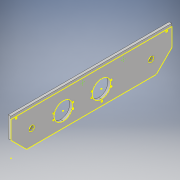
# Autodesk Inventor part: DriveTrainPlate
Saved by Autodesk Inventor 2017 (Build 210142000, 142)
## iProperties
Created: 2016-09-21
Part Number: DriveTrainPlate
Material: Generic
Document SubType Name: Modeling
Designer: RoboticsUser
Density: 1 g/cm^3
Appearance: Default
Mass: 175.92 g
Surface Area: 642.608 cm^2
Volume: 175.92 cm^3
Author: RoboticsUser
Autodesk Inventor part; units mm, degrees
ref_plane "YZ Plane" through (0, 0, 0) normal (1, 0, 0) x (0, 1, 0)
ref_plane "XZ Plane" through (0, 0, 0) normal (0, 1, 0) x (-1, 0, 0)
ref_plane "XY Plane" through (0, 0, 0) normal (0, 0, 1) x (1, 0, 0)
sketch "Sketch1" plane through (0, 0, 0) normal (1, 0, 0) x (0, 1, 0)
  line L0 (444.5, 0) -> (444.5, -2.1042)
  line L1 (0, -2.1042) -> (0, 0)
  line L2 (0, -74.1174) -> (0, -66.8433)
  line L3 (0, 0) -> (82.55, 0)
  line L4 (82.55, 0) -> (82.55, -393.7)
  line L5 (82.55, -393.7) -> (0, -393.7)
  line L6 (0, -393.7) -> (0, 0)
  point P0 (25.4, -50.8)
  point P1 (25.4, -342.9)
  dimension "d2" = 82.55
  dimension "d3" = 393.7
  dimension "d4" = 50.8
  dimension "d5" = 25.4
  dimension "d6" = 50.8
  dimension "d7" = 25.4
  constraints: 14 end point, 3 parallel, 1 horizontal, 1 perpendicular, 1 point on line
  measures "d2" distance of L4.end L5.end
  measures "d3" distance of L3.end L4.end
  measures "d4" distance from line of L3 point (25.4, -50.8)
  measures "d5" distance from line of L6 point (25.4, -50.8)
  measures "d6" distance from line of L5 point (25.4, -342.9)
  measures "d7" distance from line of L6 point (25.4, -342.9)
extrude "Extrusion1" add sketch "Sketch1" along normal blind 6.35
sketch "Sketch3" plane through (6.35, 0, 0) normal (1, 0, 0) x (0, 0, -1)
  point P0 (0, 0)
sketch "Sketch4" plane through (6.35, 0, 0) normal (1, 0, 0) x (0, 0, -1)
  point P0 (0, 0)
chamfer "Chamfer1" distance 38.1 angle 45 1 edges at (3.175, 0, 0)
chamfer "Chamfer2" distance 38.1 angle 45 1 edges at (3.175, 0, -393.7)
sketch "Sketch5" plane through (0, 0, 0) normal (-1, 0, 0) x (0, 0, 1)
  line L0 (0, 82.55) -> (-393.7, 82.55) projected
  line L1 (-355.6, 0) -> (-393.7, 38.1) projected
  line L2 (-355.6, 0) -> (-38.1, 0) projected
  line L3 (0, 38.1) -> (-38.1, 0) projected
  line L4 (0, 38.1) -> (0, 82.55) projected
  line L5 (0, 82.55) -> (-393.7, 82.55) projected
  line L6 (-393.7, 82.55) -> (-393.7, 38.1) projected
  point P0 (0, 0)
  point P1 (-342.9, 38.1)
  point P2 (-50.8, 38.1)
  dimension "d16" = 50.8
  dimension "d17" = 38.1
  dimension "d18" = 38.1
  dimension "d19" = 50.8
  measures "d16" distance from line of L6 point (-342.9, 38.1)
  measures "d17" distance from line of point (-342.9, 38.1) L2
  measures "d18" distance from line of L2 point (-50.8, 38.1)
  measures "d19" distance from line of L4 point (-50.8, 38.1)
hole "Hole1" at (0, 38.1, -342.9) at (0, 38.1, -50.8) direction (1, 0, 0) diameter 12.7254 end through all
sketch "Sketch7" plane through (0, 0, 0) normal (-1, 0, 0) x (0, 0, 1)
  line L0 (-38.1, 0) -> (-355.6, 0) projected
  line L1 (-393.7, 82.55) -> (-393.7, 38.1) projected
  line L2 (0, 38.1) -> (0, 82.55) projected
  line L3 (0, 82.55) -> (-393.7, 82.55) projected
  point P0 (0, 0)
  point P1 (-298.45, 10.0076)
  point P2 (-95.25, 10.0076)
  point P3 (-12.7, 78.8924)
  point P4 (-381, 78.8924)
  dimension "d42" = 10.0076
  dimension "d43" = 95.25
  dimension "d44" = 95.25
  dimension "d45" = 3.6576
  dimension "d46" = 12.7
  dimension "d47" = 12.7
  dimension "d82" = 3.6576
  measures "d42" distance from line of L0 point (-298.45, 10.008)
  measures "d43" distance from line of L1 point (-298.45, 10.008)
  measures "d44" distance from line of L2 point (-95.25, 10.008)
  measures "d45" distance from line of L3 point (-12.7, 78.892)
  measures "d46" distance from line of point (-12.7, 78.892) L2
  measures "d47" distance from line of L1 point (-381, 78.892)
  measures "d82" distance from line of L3 point (-381, 78.892)
hole "Hole3" at (0, 78.8924, -381) at (0, 78.8924, -12.7) direction (1, 0, 0) diameter 4.7752 end through all
sketch "Sketch8" plane through (0, 0, 0) normal (-1, 0, 0) x (0, 0, 1)
  line L0 (0, 38.1) -> (0, 82.55) projected
  line L1 (0, 82.55) -> (-393.7, 82.55) projected
  line L2 (-355.6, 0) -> (-38.1, 0) projected
  line L3 (-393.7, 38.1) -> (-393.7, 82.55) projected
  point P0 (0, 0)
  point P1 (-171.45, 78.8924)
  point P2 (-222.25, 10.0076)
  dimension "d57" = 10.0076
  dimension "d128" = 222.25
  measures "d57" distance from line of L2 point (-222.25, 10.008)
  measures "d128" distance from line of L0 point (-222.25, 10.008)
hole "Hole4" at (0, 10.0076, -222.25) direction (1, 0, 0) diameter 4.7752 end through all
sketch "Sketch10" plane through (0, 0, 0) normal (-1, 0, 0) x (0, 0, 1)
  circle A0 centre (-222.25, 36.322) radius 1.778
  circle A1 centre (-127, 36.322) radius 1.778
  line L0 (-393.7, 82.55) -> (0, 82.55) projected
  line L1 (-114.3619, 67.6125) -> (-112.4836, 67.6125)
  point P0 (0, 0)
  point P1 (-220.472, 36.322)
  point P2 (-128.778, 36.322)
  dimension "d108" = 46.228
  dimension "d109" = 46.228
  constraints: 2 end point, 2 horizontal alignment, 1 horizontal, 4 other
  measures "d108" distance from line of L0 point (-127, 36.322)
  measures "d109" distance from line of L0 point (-222.25, 36.322)
hole "Hole6" at (0, 36.322, -127) at (0, 36.322, -220.472) at (0, 36.322, -128.778) at (0, 36.322, -222.25) direction (1, 0, 0) diameter 43.18 end through all
sketch "Sketch14" plane through (6.35, 0, 0) normal (1, 0, 0) x (0, 0, -1)
  arc A0 (127.889, 57.8937) -> (127.889, 14.7503) centre (127, 36.322) ccw projected
  arc A1 (127.889, 14.7503) -> (127.889, 57.8937) centre (128.778, 36.322) ccw projected
  arc A2 (221.361, 57.8937) -> (221.361, 14.7503) centre (220.472, 36.322) ccw projected
  arc A3 (221.361, 14.7503) -> (221.361, 57.8937) centre (222.25, 36.322) ccw projected
  line L0 (127.889, 57.8937) -> (127.889, 14.7503)
  line L1 (96.03, 36.322) -> (156.5626, 36.322)
  line L2 (221.361, 57.8937) -> (221.361, 14.7503)
  line L3 (190.5646, 36.322) -> (248.6345, 36.322)
  line L4 (127.889, 36.322) -> (103.886, 36.322)
  line L5 (103.886, 36.322) -> (103.886, 43.3324)
  line L6 (103.886, 43.3324) -> (103.886, 36.322)
  line L7 (103.886, 36.322) -> (103.886, 29.3116)
  line L8 (127.889, 36.322) -> (151.892, 36.322)
  line L9 (151.892, 36.322) -> (151.892, 29.3116)
  line L10 (151.892, 36.322) -> (151.892, 43.3324)
  line L11 (221.361, 43.3324) -> (197.358, 43.3324)
  line L12 (221.361, 43.3324) -> (245.364, 43.3324)
  line L13 (221.361, 29.3116) -> (197.358, 29.3116)
  line L14 (221.361, 29.3116) -> (245.364, 29.3116)
  circle A4 centre (103.886, 29.3116) radius 1.7526
  circle A5 centre (103.886, 43.3324) radius 1.7526
  circle A6 centre (151.892, 43.3324) radius 1.7526
  circle A7 centre (151.892, 29.3116) radius 1.7526
  circle A8 centre (197.358, 43.3324) radius 1.7526
  circle A9 centre (197.358, 29.3116) radius 1.7526
  circle A10 centre (245.364, 29.3116) radius 1.7526
  circle A11 centre (245.364, 43.3324) radius 1.7526
  point P0 (0, 0)
  dimension "d113" = 24.003
  dimension "d114" = 7.0104
  dimension "d115" = 7.0104
  dimension "d116" = 24.003
  dimension "d117" = 24.003
  dimension "d118" = 24.003
  dimension "d119" = 3.5052
  dimension "d120" = 3.5052
  dimension "d121" = 3.5052
  dimension "d122" = 3.5052
  dimension "d123" = 3.5052
  constraints: 30 end point, 8 centre point, 8 coincident, 6 point on line, 5 horizontal, 3 perpendicular, 3 vertical, 1 collinear, 1 midpoint
  measures "d113" distance of L4.start L4.end
  measures "d114" distance of L4.end L5.end
  measures "d115" distance of L4.end L7.end
  measures "d116" distance of L4.start L8.end
  measures "d117" distance of L11.start L11.end
  measures "d118" distance of L11.start L12.end
  measures "d119" diameter of A4
  measures "d120" diameter of A5
  measures "d121" diameter of A6
  measures "d122" diameter of A7
  measures "d123" diameter of A8
extrude "Extrusion2" cut sketch "Sketch14" against normal blind 25.4 contours A4 | A5 | A6 | A7 | A8 | A9 | A10 | A11
sketch "Sketch15" plane through (6.35, 0, 0) normal (1, 0, 0) x (0, 0, -1)
  circle A0 centre (245.364, 29.3116) radius 1.7526 projected
  circle A1 centre (197.358, 43.3324) radius 1.7526 projected
  circle A2 centre (151.892, 43.3324) radius 1.7526 projected
  circle A3 centre (103.886, 29.3116) radius 1.7526 projected
  circle A4 centre (103.886, 43.3324) radius 1.7526 projected
  circle A5 centre (151.892, 29.3116) radius 1.7526 projected
  circle A6 centre (197.358, 29.3116) radius 1.7526 projected
  circle A7 centre (245.364, 43.3324) radius 1.7526 projected
  arc A8 (127.889, 14.7503) -> (127.889, 57.8937) centre (128.778, 36.322) ccw projected
  arc A9 (127.889, 57.8937) -> (127.889, 14.7503) centre (127, 36.322) ccw projected
  arc A10 (221.361, 14.7503) -> (221.361, 57.8937) centre (222.25, 36.322) ccw projected
  arc A11 (221.361, 57.8937) -> (221.361, 14.7503) centre (220.472, 36.322) ccw projected
  circle A12 centre (222.25, 10.0076) radius 2.3876 projected
  circle A13 centre (381, 78.8924) radius 2.3876 projected
  circle A14 centre (12.7, 78.8924) radius 2.3876 projected
  circle A15 centre (342.9, 38.1) radius 6.3627 projected
  circle A16 centre (50.8, 38.1) radius 6.3627 projected
  line L0 (393.7, 38.1) -> (355.6, 0) projected
  line L1 (393.7, 38.1) -> (393.7, 82.55) projected
  line L2 (393.7, 82.55) -> (0, 82.55) projected
  line L3 (0, 82.55) -> (0, 38.1) projected
  line L4 (38.1, 0) -> (0, 38.1) projected
  line L5 (38.1, 0) -> (355.6, 0) projected
  point P0 (0, 0)
  point P1 (175.7134, 71.7703)
  point P2 (275.9443, 71.7703)
thicken "Thicken1" operation add thickness 6.35 both sides no extend neighbours yes toward (0, 1, 0) faces at (2.1167, 82.55, -131.2333)
body "Solid1"
